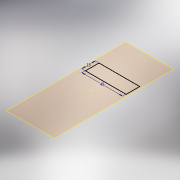
# Autodesk Inventor part: HTD-5M-belt-clamp
Saved by Autodesk Inventor 2016 (Build 200138000, 138)
## iProperties
Created: 2015-05-09
Part Number: HTD-5M-belt-clamp
Material: Aluminum 6061
Document SubType Name: Modeling
Designer: ax
Mass: 3.645 g
Surface Area: 15.9 cm^2
Volume: 1.35 cm^3
Density: 2.7 g/cm^3
Appearance: Aluminum - Flat
Author: ax
Autodesk Inventor part; units mm, degrees
ref_plane "YZ Plane" through (0, 0, 0) normal (1, 0, 0) x (0, 1, 0)
ref_plane "XZ Plane" through (0, 0, 0) normal (0, 1, 0) x (-1, 0, 0)
ref_plane "XY Plane" through (0, 0, 0) normal (0, 0, 1) x (1, 0, 0)
ref_plane "Work Plane1" through (0, 0, 0) normal (0, 0, 1) x (1, 0, 0)
sketch "Sketch2" plane through (0, 0, 0) normal (0, 0, 1) x (1, 0, 0)
  line L0 (22.5, 31) -> (-22.5, 31)
  line L1 (-22.5, 31) -> (-22.5, 16)
  line L2 (-22.5, 16) -> (22.5, 16)
  line L3 (22.5, 16) -> (22.5, 31)
  point P0 (0, 0)
  dimension "d1" = 15
  dimension "d4" = 45
  dimension "d5" = 22.5
  dimension "d6" = 31
  constraints: 8 end point, 2 parallel, 1 horizontal, 1 perpendicular
  measures "d1" distance of L1.end L0.end
  measures "d4" distance between parallel lines of L1 L3
  measures "d5" distance from line of point (0, 0) L3
  measures "d6" distance from line of point (0, 0) L0
extrude "Extrusion1" add sketch "Sketch2" along normal blind 2
body "Solid1"
